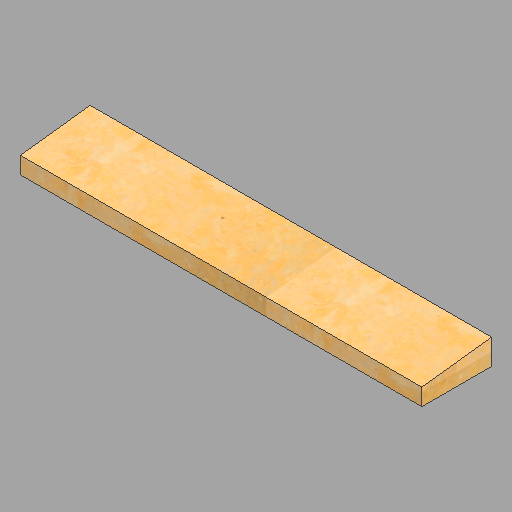
# Autodesk Inventor part: Sill
Saved by Autodesk Inventor 2023 (Build 270158030, 158C)
## iProperties
RuleStatus: InUse
Created: 2022-06-21
Part Number: Sill
Material: Granite, Cut, Polished
Document SubType Name: Modeling
Designer: awelt
Mass: 43346.3 g
Surface Area: 6873.33 cm^2
Volume: 16054.2 cm^3
Density: 2.7 g/cm^3
Appearance: Amber Select
AfterDocSave0: Convert in3 volume to ft3
in3 to ft3: 0.0
TEST: 0.0
Author: awelt
Autodesk Inventor part; units mm, degrees
ref_plane "YZ Plane" through (0, 0, 0) normal (1, 0, 0) x (0, 1, 0)
ref_plane "XZ Plane" through (0, 0, 0) normal (0, 1, 0) x (-1, 0, 0)
ref_plane "XY Plane" through (0, 0, 0) normal (0, 0, 1) x (1, 0, 0)
sketch "Sketch1" plane through (0, 0, 0) normal (1, 0, 0) x (0, 1, 0)
  line L0 (0, 0) -> (76.2, 0)
  line L1 (0, 0) -> (0, 209.55)
  line L2 (0, 209.55) -> (50.8, 209.55)
  line L3 (50.8, 209.55) -> (76.2, 0)
  dimension "d0" = 76.2
  dimension "d1" = 209.55
  dimension "d2" = 50.8
  constraints: 8 end point, 1 horizontal, 1 perpendicular, 1 vertical
  measures "d0" distance of L0.start L0.end
  measures "d1" distance of L0.start L1.end
  measures "d2" distance of L1.end L2.end
extrude "Extrusion1" add sketch "Sketch1" along normal blind 1206.5
body "Solid1"
